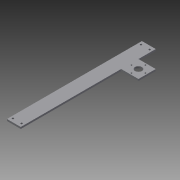
# Autodesk Inventor part: Cim Mount
Saved by Autodesk Inventor 2013 (Build 170138000, 138)
## iProperties
Created: 2013-01-24
Part Number: Cim Mount
Material: Generic
Document SubType Name: Modeling
Designer: actoennies
Density: 1 g/cm^3
Author: actoennies
Autodesk Inventor part; units mm, degrees
ref_plane "YZ Plane" through (0, 0, 0) normal (1, 0, 0) x (0, 1, 0)
ref_plane "XZ Plane" through (0, 0, 0) normal (0, 1, 0) x (-1, 0, 0)
ref_plane "XY Plane" through (0, 0, 0) normal (0, 0, 1) x (1, 0, 0)
sketch "Sketch1" plane through (0, 0, 0) normal (0, 1, 0) x (-1, 0, 0)
  line L0 (0, 0) -> (0, 63.5)
  line L1 (0, 63.5) -> (-63.5, 63.5)
  line L2 (-63.5, 63.5) -> (-63.5, 127)
  line L3 (-63.5, 127) -> (0, 127)
  line L4 (0, 127) -> (0, 495.3)
  line L5 (0, 495.3) -> (50.8, 495.3)
  line L6 (50.8, 495.3) -> (50.8, 0)
  line L7 (50.8, 0) -> (0, 0)
  circle A0 centre (-31.75, 95.25) radius 25.4 construction
  circle A1 centre (-31.75, 120.65) radius 2.5527
  circle A2 centre (-6.35, 95.25) radius 2.5527
  circle A3 centre (-57.15, 95.25) radius 2.5527
  circle A4 centre (-31.75, 69.85) radius 2.5527
  dimension "d1" = 63.5
  dimension "d2" = 63.5
  dimension "d3" = 63.5
  dimension "d4" = 368.3
  dimension "d5" = 50.8
  dimension "d6" = 50.8
  dimension "d7" = 5.1054
  dimension "d8" = 5.1054
  dimension "d9" = 5.1054
  dimension "d10" = 5.1054
  constraints: 16 end point, 5 centre point, 4 perpendicular, 4 point on circle, 3 parallel, 1 vertical
  measures "d1" distance of L0.start L0.end
  measures "d2" distance of L0.end L1.end
  measures "d3" distance of L1.end L2.end
  measures "d4" distance of L3.end L4.end
  measures "d5" distance of L4.end L5.end
  measures "d6" diameter of A0
  measures "d7" diameter of A1
  measures "d8" diameter of A2
  measures "d9" diameter of A3
  measures "d10" diameter of A4
extrude "Extrusion1" add sketch "Sketch1" along normal blind 6.35
sketch "Sketch2" plane through (0, 6.35, 0) normal (0, 1, 0) x (1, 0, 0)
  circle A0 centre (31.75, -95.25) radius 12.7
  dimension "d13" = 25.4
  constraints: 1 centre point
  measures "d13" diameter of A0
extrude "Extrusion2" cut sketch "Sketch2" against normal blind 6.35
sketch "Sketch3" plane through (0, 6.35, 0) normal (0, 1, 0) x (1, 0, 0)
  line L0 (0, -63.5) -> (0, 0) projected
  line L1 (0, 0) -> (-50.8, 0) projected
  line L2 (-50.8, 0) -> (-50.8, -495.3) projected
  line L3 (-50.8, -495.3) -> (0, -495.3) projected
  line L4 (0, -495.3) -> (0, -127) projected
  circle A0 centre (-41.275, -12.7) radius 3.3782
  circle A1 centre (-9.525, -12.7) radius 3.3782
  circle A2 centre (-41.275, -482.6) radius 3.3782
  circle A3 centre (-9.525, -482.6) radius 3.3782
  dimension "d16" = 6.7564
  dimension "d17" = 6.7564
  dimension "d18" = 6.7564
  dimension "d19" = 6.7564
  dimension "d20" = 12.7
  dimension "d21" = 12.7
  dimension "d22" = 9.525
  dimension "d23" = 9.525
  dimension "d24" = 12.7
  dimension "d25" = 12.7
  dimension "d26" = 9.525
  dimension "d27" = 9.525
  constraints: 4 centre point
  measures "d16" diameter of A0
  measures "d17" diameter of A1
  measures "d18" diameter of A2
  measures "d19" diameter of A3
  measures "d20" distance from line of L3 A2.centre
  measures "d21" distance from line of L3 A3.centre
  measures "d22" distance from line of L4 A3.centre
  measures "d23" distance from line of L2 A2.centre
  measures "d24" distance from line of L1 A1.centre
  measures "d25" distance from line of L1 A0.centre
  measures "d26" distance from line of L2 A0.centre
  measures "d27" distance from line of L0 A1.centre
extrude "Extrusion3" cut sketch "Sketch3" against normal blind 25.4
body "Solid1"
